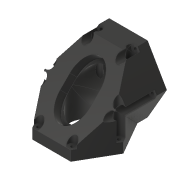
# Autodesk Inventor part: TARM01
Saved by Autodesk Inventor 2017 (Build 210142000, 142)
## iProperties
Created: 2018-10-11
Part Number: TARM01
Material: ABS Plastic
Document SubType Name: Modeling
Designer: Zach
Density: 1.06 g/cm^3
Appearance: Smooth - Black
Author: Zach
Autodesk Inventor part; units mm, degrees
ref_plane "YZ Plane" through (0, 0, 0) normal (1, 0, 0) x (0, 1, 0)
ref_plane "XZ Plane" through (0, 0, 0) normal (0, 1, 0) x (-1, 0, 0)
ref_plane "XY Plane" through (0, 0, 0) normal (0, 0, 1) x (1, 0, 0)
sketch "Sketch38" plane through (0, 0, 0) normal (0, 0, 1) x (1, 0, 0)
  line L0 (57.5, 0) -> (28.75, -49.796461)
  line L1 (28.75, -49.796461) -> (-28.75, -49.796461)
  line L2 (-28.75, -49.796461) -> (-57.5, 0)
  line L3 (-57.5, 0) -> (-28.75, 49.796461)
  line L4 (-28.75, 49.796461) -> (28.75, 49.796461)
  line L5 (28.75, 49.796461) -> (57.5, 0)
  circle A0 centre (-51, 0) radius 2.5
  circle A1 centre (51, 0) radius 2.5 construction
  line L6 (-51, 0) -> (51, 0) construction
  circle A2 centre (-25.5, -44.167296) radius 2.5
  circle A3 centre (25.5, -44.167296) radius 2.5
  circle A4 centre (51, 0) radius 2.5
  circle A5 centre (25.5, 44.167296) radius 2.5
  circle A6 centre (-25.5, 44.167296) radius 2.5
  circle A7 centre (0, 0) radius 22.5
  dimension "d163" = 115
  dimension "d164" = 5
  dimension "d165" = 5
  dimension "d166" = 102
  dimension "d169" = 360
  dimension "d171" = 45
  constraints: 14 end point, 8 centre point, 3 coincident, 1 horizontal, 1 horizontal alignment, 1 midpoint, 26 other
  measures "d163" distance of L0.start L2.end
  measures "d164" diameter of A0
  measures "d165" diameter of A1
  measures "d166" distance of L6.start L6.end
  measures "d171" diameter of A7
extrude "Extrusion31" add sketch "Sketch38" along normal blind 150
sketch "Sketch39" plane through (-28.75, -49.796461, 0) normal (0, -1, 0) x (1, 0, 0)
  line L0 (57.5, 150) -> (86.25, 100.203539)
  line L1 (86.25, 100.203539) -> (57.5, 50.407079)
  line L2 (57.5, 50.407079) -> (0, 50.407079)
  line L3 (0, 50.407079) -> (-28.75, 100.203539)
  line L4 (-28.75, 100.203539) -> (0, 150)
  line L5 (0, 150) -> (57.5, 150)
  line L6 (0, 150) -> (57.5, 150)
  line L7 (6.25, 150) -> (51.25, 150)
  line L8 (86.25, 0) -> (86.25, 150)
  line L9 (-28.75, 0) -> (-28.75, 150)
  line L10 (57.5, 150) -> (0, 150)
  line L11 (0, 150) -> (-28.75, 150)
  line L12 (-28.75, 150) -> (-28.75, 100.203539)
  line L13 (-28.75, 100.203539) -> (0, 150)
  line L14 (86.25, 150) -> (57.5, 150)
  line L15 (86.25, 150) -> (57.5, 150)
  line L16 (57.5, 150) -> (86.25, 100.203539)
  line L17 (86.25, 150) -> (86.25, 100.203539)
  point P0 (28.75, 0)
  point P1 (28.75, 100.203539)
  point P2 (28.75, 150)
  constraints: 24 end point, 2 collinear, 2 midpoint, 2 perpendicular, 2 point on line, 1 horizontal alignment, 13 other
extrude "Extrusion32" cut sketch "Sketch39" against normal through all contours L14 L8 L0 | L4 L9 L11
extrude "Extrusion33" add sketch "Sketch39" against normal through all contours L0 L1 L2 L3 L4 L5
sketch "Sketch40" plane through (0, 0, 0) normal (0, 0, -1) x (-1, 0, 0)
  circle A0 centre (0, 0) radius 22.5 projected
extrude "Extrusion34" cut sketch "Sketch40" against normal through all
chamfer "Chamfer4" distance 85 angle 45 1 edges at (0, 49.7965, 150)
ref_plane "Work Plane1" through (-28.75, -34.796461, 0) normal (0, -1, 0) x (1, 0, 0)
sketch "Sketch41" plane through (-28.75, -34.796461, 0) normal (0, -1, 0) x (1, 0, 0)
  line L0 (57.5, 50.407079) -> (86.25, 100.203539)
  line L1 (86.25, 100.203539) -> (57.5, 150)
  line L2 (0, 150) -> (57.5, 150)
  line L3 (0, 150) -> (-28.75, 100.203539)
  line L4 (-28.75, 100.203539) -> (0, 50.407079)
  line L5 (0, 0) -> (0, 50.407079)
  line L6 (57.5, 0) -> (0, 0)
  line L7 (57.5, 0) -> (57.5, 50.407079) construction
  circle A0 centre (-22.25, 100.203539) radius 2.5
  line L8 (0, 150) -> (-28.75, 100.203539)
  line L9 (-28.75, 100.203539) -> (86.25, 100.203539) construction
  circle A1 centre (3.25, 56.036244) radius 2.5
  circle A2 centre (54.25, 56.036244) radius 2.5
  circle A3 centre (79.75, 100.203539) radius 2.5
  circle A4 centre (54.25, 144.370835) radius 2.5
  circle A5 centre (3.25, 144.370835) radius 2.5
  point P0 (28.75, 0)
  point P1 (28.75, 100.203539)
  dimension "d185" = 5
  dimension "d186" = 51
  dimension "d189" = 360
  constraints: 6 centre point, 2 end point, 1 horizontal, 1 midpoint, 1 point on line, 13 other
  measures "d185" diameter of A0
  measures "d186" distance of A0.centre point (28.75, 100.204)
extrude "Extrusion35" cut sketch "Sketch41" along normal through all both and the other way through all
sketch "Sketch42" plane through (-28.75, -34.796461, 0) normal (0, -1, 0) x (1, 0, 0)
  arc A0 (-21.737493, 102.650443) -> (-19.874666, 99.423931) centre (-22.25, 100.203539) ccw construction
  circle A1 centre (-22.25, 100.203539) radius 2.5 construction
  circle A2 centre (-22.25, 100.203539) radius 6.5
  circle A3 centre (79.75, 100.203539) radius 2.5
  line L0 (-22.25, 100.203539) -> (79.75, 100.203539) construction
  circle A4 centre (3.25, 56.036244) radius 6.5
  circle A5 centre (54.25, 56.036244) radius 6.5
  circle A6 centre (79.75, 100.203539) radius 6.5
  circle A7 centre (54.25, 144.370835) radius 6.5
  circle A8 centre (3.25, 144.370835) radius 6.5
  point P0 (28.75, 0)
  point P1 (28.75, 100.203539)
  dimension "d193" = 13
  dimension "d196" = 360
  constraints: 6 centre point, 2 end point, 1 coincident, 1 horizontal, 1 midpoint, 13 other
  measures "d193" diameter of A2
extrude "Extrusion36" cut sketch "Sketch42" against normal through all contours A2 | A3 | A4 | A5 | A6 | A7 | A8
sketch "Sketch44" plane through (-28.75, -49.796461, 0) normal (0, -1, 0) x (1, 0, 0)
  circle A0 centre (79.75, 100.203539) radius 2.5 construction
  line L0 (79.75, 100.203539) -> (-22.25, 100.203539) construction
  circle A1 centre (-22.25, 100.203539) radius 2.5 construction
  circle A2 centre (28.75, 100.203539) radius 22.5
  point P0 (28.75, 0)
  dimension "d200" = 45
  constraints: 3 end point, 1 centre point, 1 horizontal, 1 midpoint
  measures "d200" diameter of A2
extrude "Extrusion37" cut sketch "Sketch44" against normal through all
sketch "Sketch45" plane through (-28.75, 49.796461, 65) normal (0, 0.7071068, 0.7071068) x (1, 0, 0)
  ellipse E0 centre (28.75, -49.785323) end of major axis (28.75, -81.605128) minor radius 22.5 (50.034071, -60.104076) -> (7.465929, -60.104076) ccw
  ellipse E1 centre (28.75, -70.42283) end of major axis (28.75, -102.242635) minor radius 22.5 (7.465929, -60.104076) -> (50.034071, -60.104076) ccw
  line L0 (6.25, -49.785323) -> (6.25, -70.42283)
  line L1 (51.25, -49.785323) -> (51.25, -70.42283)
  line L2 (7.465929, -60.104076) -> (6.25, -60.104076)
  point P0 (28.75, 10.750526)
  constraints: 5 vertical, 4 end point, 6 other
extrude "Extrusion38" cut sketch "Sketch45" against normal blind 15
fillet "Fillet1" radius 15 2 edges at (14.6925, -17.0405, 83.163) (-14.6925, -17.0405, 83.163)
sketch "Sketch46" plane through (-28.75, -34.796461, 0) normal (0, 1, 0) x (1, 0, 0)
  arc A0 (-25.5, -105.832704) -> (-25.5, -94.574374) centre (-22.25, -100.203539) ccw
  line L0 (-22.25, -93.703539) -> (-37.25, -93.703539)
  line L1 (-37.25, -93.703539) -> (-37.25, -106.703539)
  line L2 (-37.25, -106.703539) -> (-22.25, -106.703539)
  arc A1 (-23.947342, -106.478014) -> (-17.664817, -95.59636) centre (-22.25, -100.203539) ccw
  arc A2 (75.164817, -95.59636) -> (81.447342, -106.478014) centre (79.75, -100.203539) ccw
  arc A3 (86.25, -100.203539) -> (75.164817, -95.59636) centre (79.75, -100.203539) ccw
  line L3 (79.75, -93.703539) -> (94.75, -93.703539)
  line L4 (94.75, -93.703539) -> (94.75, -106.703539)
  line L5 (94.75, -106.703539) -> (79.75, -106.703539)
  point P0 (28.75, 0)
  dimension "d206" = 15
  dimension "d207" = 15
  constraints: 12 end point, 4 point on circle, 4 tangent, 3 horizontal, 3 perpendicular
  measures "d206" distance of L0.start L0.end
  measures "d207" distance of L3.start L3.end
extrude "Extrusion39" cut sketch "Sketch46" along normal through all
sketch "Sketch48" plane through (0, 0, 0) normal (0, 0, -1) x (-1, 0, 0)
  circle A0 centre (0, 0) radius 22.5
  circle A1 centre (25.5, 44.167296) radius 2.5
  circle A2 centre (-25.5, 44.167296) radius 2.5
  circle A3 centre (-51, 0) radius 2.5
  circle A4 centre (-25.5, -44.167296) radius 2.5
  circle A5 centre (25.5, -44.167296) radius 2.5
  circle A6 centre (51, 0) radius 2.5
  line L0 (-57.5, 0) -> (-28.75, -49.796461)
  line L1 (-28.75, -49.796461) -> (28.75, -49.796461)
  line L2 (28.75, -49.796461) -> (57.5, 0)
  line L3 (57.5, 0) -> (28.75, 49.796461)
  line L4 (28.75, 49.796461) -> (-28.75, 49.796461)
  line L5 (-28.75, 49.796461) -> (-57.5, 0)
extrude "Extrusion40" cut sketch "Sketch48" against normal blind 35 contours A0 | A1 | A2 | A3 | A4 | A5 | A6 | L5 L4 L3 L2 L1 L0
ref_plane "Work Plane2" through (0, 0, 50) normal (0, 0, -1) x (-1, 0, 0)
sketch "Sketch49" plane through (0, 0, 50) normal (0, 0, -1) x (-1, 0, 0)
  circle A0 centre (-25.5, 44.167296) radius 2.5
  circle A1 centre (-25.5, 44.167296) radius 6.5
  circle A2 centre (25.5, 44.167296) radius 6.5
  circle A3 centre (51, 0) radius 6.5
  circle A4 centre (25.5, -44.167296) radius 6.5
  circle A5 centre (-25.5, -44.167296) radius 6.5
  circle A6 centre (-51, 0) radius 6.5
  point P0 (0, 0)
  dimension "d213" = 13
  dimension "d216" = 360
  constraints: 6 centre point, 1 coincident, 13 other
  measures "d213" diameter of A1
extrude "Extrusion41" cut sketch "Sketch49" against normal through all contours A0 | A1 | A2 | A3 | A6
body "Solid3"
